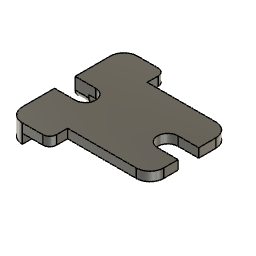
Phone Stand V1 v4 v2 (Autodesk Fusion 360 design; units mm, degrees)
Autodesk Fusion 360 part; units mm, degrees
note: some values were not read from the file. Set by a fixed rule: which sketch regions a step uses.
sketch "Phone Stand Backing" plane through (0, 0, 0) normal (0, 0, 1) x (1, 0, 0)
  line L0 (-10, 0) -> (-163, 0)
  line L1 (-173, -10) -> (-173, -77.6)
  line L2 (-163, -87.6) -> (-10, -87.6)
  line L3 (-20, -51.3) -> (0, -51.3)
  line L4 (-20, -36.3) -> (0, -36.3)
  arc A0 (-20, -36.3) -> (-20, -51.3) centre (-20, -43.8) ccw
  line L5 (-148, -38.8) -> (-65, -38.8)
  line L6 (-65, -48.8) -> (-148, -48.8)
  arc A1 (-148, -38.8) -> (-148, -48.8) centre (-148, -43.8) ccw
  arc A2 (-65, -48.8) -> (-65, -38.8) centre (-65, -43.8) ccw
  line L7 (-148, -24.8) -> (-65, -24.8)
  line L8 (-65, -14.8) -> (-148, -14.8)
  arc A3 (-148, -14.8) -> (-148, -24.8) centre (-148, -19.8) ccw
  arc A4 (-65, -24.8) -> (-65, -14.8) centre (-65, -19.8) ccw
  line L9 (-148, -62.8) -> (-65, -62.8)
  arc A5 (-148, -62.8) -> (-148, -72.8) centre (-148, -67.8) ccw
  line L10 (-65, -72.8) -> (-148, -72.8)
  arc A6 (-65, -72.8) -> (-65, -62.8) centre (-65, -67.8) ccw
  arc A7 (-173, -77.6) -> (-163, -87.6) centre (-163, -77.6) ccw
  arc A8 (-163, 0) -> (-173, -10) centre (-163, -10) ccw
  arc A9 (0, -10) -> (-10, 0) centre (-10, -10) ccw
  arc A10 (-10, -87.6) -> (0, -77.6) centre (-10, -77.6) ccw
  line L11 (-47.25, -70) -> (-47.25, -17.6)
  line L12 (-40.25, -17.6) -> (-40.25, -70)
  arc A11 (-47.25, -70) -> (-40.25, -70) centre (-43.75, -70) ccw
  arc A12 (-40.25, -17.6) -> (-47.25, -17.6) centre (-43.75, -17.6) ccw
  line L13 (0, -77.6) -> (0, -51.3)
  line L14 (0, -36.3) -> (0, -10)
  dimension "d3" = 15
  dimension "d4" = 20
  dimension "d5" = 10
  dimension "d6" = 10
  dimension "d7" = 25
  dimension "d8" = 45
  dimension "d9" = 19
  dimension "d10" = 10
  dimension "d11" = 10
  dimension "d12" = 14
  dimension "d13" = 14.8
  dimension "d14" = 65
  dimension "d15" = 10
  dimension "d16" = 173
  dimension "d17" = 10
  dimension "d18" = 10
  dimension "d19" = 10
  dimension "d20" = 36.3
  dimension "d21" = 36.3
  dimension "d22" = 10
  dimension "d23" = 10
  dimension "d24" = 14.8
  dimension "d25" = 83
  dimension "d26" = 25
  dimension "d27" = 7
  dimension "d29" = 52.4
  dimension "d31" = 17.6
  dimension "d32" = 17.6
  dimension "d33" = 23.75
  dimension "d70" = 3.5
  constraint horizontal L0
  constraint vertical L1
  constraint horizontal L2
  constraint vertical L13
  constraint tangent L3 A0
  constraint perpendicular L3 L13
  constraint coincident L4.end L13
  constraint tangent L4 A0
  constraint perpendicular L4 L13
  constraint tangent L5 A2
  constraint tangent L6 A1
  constraint tangent L7 A4
  constraint tangent L8 A3
  constraint parallel L7 L8
  constraint tangent L1 A7
  constraint tangent L2 A7
  constraint coincident origin L0
  constraint coincident origin L13
  constraint tangent L0 A9
  constraint tangent A9 L13
  constraint parallel L7 L9
  constraint parallel L6 L10
  constraint tangent L7 A3
  constraint tangent L0 A8
  constraint tangent L1 A8
  constraint tangent A10 L13
  constraint tangent L2 A10
  constraint tangent L9 A5
  constraint tangent L10 A6
  constraint tangent L9 A6
  constraint tangent A5 L10
  constraint tangent L11 A12
  constraint coincident L12.end A11
  constraint tangent L12 A11
  constraint coincident L12 A11.end
  constraint tangent L12 A12
  constraint tangent L11 A11
  constraint collinear L13 L14
  measures "d3" diameter of A0
  measures "d4" distance of A0.centre L13
  measures "d5" diameter of A1
  measures "d6" diameter of A2
  measures "d7" distance of L1 A1.centre
  measures "d8" distance of A0.centre A2.centre
  measures "d9" distance of L5.start A3.centre
  measures "d10" diameter of A3
  measures "d11" diameter of A4
  measures "d12" distance of L5 L7
  measures "d13" distance of L0 L8
  measures "d14" distance of A4.centre L13
  measures "d15" radius of A7
  measures "d16" distance of L1 L13
  measures "d17" radius of A9
  measures "d18" distance of L5 L6
  measures "d19" radius of A8
  measures "d20" distance of L2 L3
  measures "d21" distance of L0 L4
  measures "d22" radius of A10
  measures "d23" distance of L9 L10
  measures "d24" distance of L2 L10
  measures "d25" distance of A5.end L10.start
  measures "d26" distance of L1 A5.centre
  measures "d27" diameter of A11
  measures "d29" distance of A11.centre A12.centre
  measures "d31" distance of L0 A12.centre
  measures "d32" distance of L2 A11.centre
  measures "d33" horizontal distance of A0.centre A11.centre
  measures "d70" radius of A12
sketch "Phone Stand Base" plane through (0, 0, 0) normal (0, 0, 1) x (1, 0, 0)
  line L0 (10, 0) -> (60, 0)
  line L1 (60, 58) -> (10, 58)
  line L2 (90, 20.5) -> (90, -3)
  line L3 (80, -13) -> (65, -13)
  line L4 (65, 71) -> (80, 71)
  line L5 (75, 20.5) -> (90, 20.5)
  line L6 (75, 35.5) -> (90, 35.5)
  arc A0 (75, 35.5) -> (75, 20.5) centre (75, 28) ccw
  line L7 (60, -8) -> (60, 0)
  line L8 (60, 58) -> (60, 66)
  line L9 (90, 61) -> (90, 35.5)
  line L10 (90, 20.5) -> (90, -3)
  arc A1 (80, -13) -> (90, -3) centre (80, -3) ccw
  arc A2 (90, 61) -> (80, 71) centre (80, 61) ccw
  line L11 (80, 20.5) -> (80, -13)
  line L12 (80, 35.5) -> (80, 71)
  arc A3 (0, 10) -> (10, 0) centre (10, 10) ccw
  arc A4 (10, 58) -> (0, 48) centre (10, 48) ccw
  arc A5 (60, -8) -> (65, -13) centre (65, -8) ccw
  arc A6 (65, 71) -> (60, 66) centre (65, 66) ccw
  line L13 (15, 20.5) -> (0, 20.5)
  line L14 (15, 35.5) -> (0, 35.5)
  arc A7 (15, 20.5) -> (15, 35.5) centre (15, 28) ccw
  line L15 (0, 48) -> (0, 35.5)
  line L16 (0, 20.5) -> (0, 10)
  point P0 (0, 58)
  point P1 (60, -13)
  point P2 (60, 71)
  point P3 (90, 71)
  dimension "d37" = 60
  dimension "d38" = 58
  dimension "d44" = 15
  dimension "d45" = 13
  dimension "d46" = 10
  dimension "d47" = 10
  dimension "d48" = 10
  dimension "d49" = 20
  dimension "d50" = 13
  dimension "d51" = 15
  dimension "d52" = 35.5
  dimension "d53" = 10
  dimension "d54" = 10
  dimension "d55" = 5
  dimension "d56" = 5
  dimension "d63" = 15
  dimension "d64" = 15
  dimension "d65" = 22.5
  constraint horizontal L0
  constraint horizontal L1
  constraint vertical L15
  constraint horizontal L3
  constraint vertical L7
  constraint horizontal L4
  constraint vertical L9
  constraint coincident L2.start L9
  constraint tangent L6 A0
  constraint perpendicular L5 L9
  constraint perpendicular L6 L9
  constraint tangent L5 A0
  constraint collinear L7 L8
  constraint collinear L9 L10
  constraint tangent L2 A1
  constraint tangent L3 A1
  constraint coincident P3 L4
  constraint coincident P3 L9
  constraint tangent L4 A2
  constraint tangent L9 A2
  constraint coincident L5 L11.start
  constraint coincident L3 A1.start
  constraint perpendicular L3 L11
  constraint coincident L6 L12.start
  constraint coincident L4 A2.end
  constraint perpendicular L4 L12
  constraint collinear L11 L12
  constraint coincident origin L0
  constraint coincident origin L15
  constraint tangent L0 A3
  constraint tangent A3 L15
  constraint coincident P0 L1
  constraint coincident P0 L15
  constraint tangent L1 A4
  constraint tangent A4 L15
  constraint coincident P1 L3
  constraint coincident P1 L7
  constraint tangent L3 A5
  constraint tangent L7 A5
  constraint coincident P2 L4
  constraint coincident P2 L8
  constraint tangent L4 A6
  constraint tangent L8 A6
  constraint coincident L13.end L15
  constraint tangent L13 A7
  constraint perpendicular L13 L15
  constraint tangent L14 A7
  constraint perpendicular L14 L15
  constraint collinear L15 L16
  measures "d37" distance of origin L0.end
  measures "d38" distance of origin P0
  measures "d44" diameter of A0
  measures "d45" distance of L0.end P1
  measures "d46" radius of A1
  measures "d47" radius of A2
  measures "d48" distance of L2 L11
  measures "d49" distance of P1 L3.start
  measures "d50" distance of L1.start P2
  measures "d51" horizontal distance of A0.centre L6.end
  measures "d52" distance of L4 L6
  measures "d53" radius of A3
  measures "d54" radius of A4
  measures "d55" radius of A5
  measures "d56" radius of A6
  measures "d63" diameter of A7
  measures "d64" distance of L13.start L13.end
  measures "d65" distance of L1 L14
extrude "Extrude2" add sketch "Phone Stand Base" along normal blind 10 contours L0 L1 L3 L4 L5 L6 A0 L7 L8 L11 L12 A3 A4 A5 A6 L13 L14 A7 L15 L16
extrude "Extrude3" add sketch "Phone Stand Base" along normal blind 17 contours L2 L5 L10 A1 L11 | L6 L9 A2 L12
fillet "Fillet1" radius 5 2 edges at (85, 20.5, 17) (85, 35.5, 17)
move_body "Move2" bodies 1 to x (1, 0, 0) y (0, 1, 0) z (0, 0, 1) at (-200, 0, -120)
move_body "Move3" bodies 1 to x (1, 0, 0) y (0, 1, 0) z (0, 0, 1) at (0, -73.75, 0)
move_body "Move4" bodies 1 to x (1, 0, 0) y (0, 1, 0) z (0, 0, 1) at (0, 0, -14.5)
move_body "Move5" bodies 1 to x (1, 0, 0) y (0, 1, 0) z (0, 0, 1) at (-21, 0, 0)
move_body "Move6" bodies 1 to x (-1, 0, 0) y (0, 1, 0) z (0, 0, -1) at (-442, 0, -139)
move_body "Move7" bodies 1 to x (1, 0, 0) y (0, 1, 0) z (0, 0, 1) at (0, 0, 4)
extrude "Extrude4" cut 1 faces at (-271, -33.9233, -0.5) along direction (0, 0, -1) blind 3
extrude "Extrude6" cut 1 faces at (-271, -33.9233, -3.5) along direction (0, 0, -1) blind 0.4
